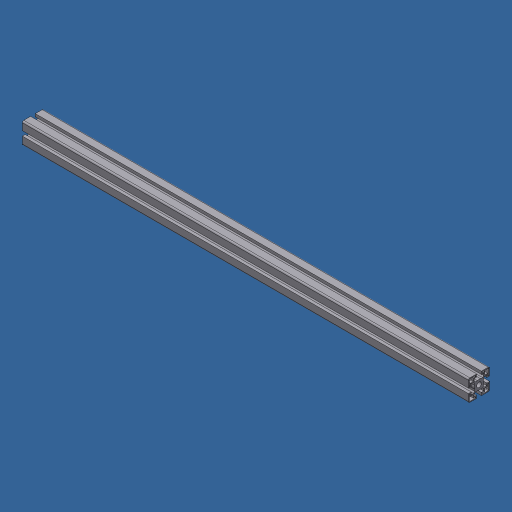
# Autodesk Inventor part: BAR, EXTRUDED ALUM, 45MMX45MM, BOSCH
Saved by Autodesk Inventor 2024.3 (Build 283343000, 343)
## iProperties
Manager: _
Category: _
RuleStatus: InUse
Shininess: 64.0
Angle Display Precision: 2
Document Length Units: 11269
Document Angle Units: 11279
Document Time Units: 11290
Document Mass Units: 11286
Document Length Units Precision: 3
Document Angle Units Precision: 2
Part Number: BAR, EXTRUDED ALUM, 45MMX45MM, BOSCH
Material: Aluminum, 6061-T6
Document SubType Name: Modeling
Created: 2019-07-31
Designer: -
Manufacturer: Standard
Standards Organization: Custom
Checked By: 00
Engr Approved By: R
User Status: Work In Proces
Description: BAR, EXTRUDED ALUM, 45MMX45MM, BOSCH
Density: 2.71 g/cm^3
Mass: 2044.87 g
Surface Area: 5623.1 cm^2
Volume: 754.565 cm^3
Mfg Approved By: -
Appearance: Aluminum (Flat)
BeforeDocSave0: Mass
BeforeDocSave1: PartFinishTrigger
Density: 0.0
Volumn: 0.0
Area: 0.0
PropertySet Name: Model Information
Control State: 0
Master: False
Checked Out: False
CN_MASS: 5.93
CN_SERVICEABLE: _
CL_runCount: 0
FIRST_DESCRIPTION: _
SECOND_DESCRIPTION: _
THIRD_DESCRIPTION: _
Revision Number: A
Subject: _
Author: -
Keywords: -
Autodesk Inventor part; units mm, degrees
ref_plane "YZ Plane" through (0, 0, 0) normal (1, 0, 0) x (0, 1, 0)
ref_plane "XZ Plane" through (0, 0, 0) normal (0, 1, 0) x (-1, 0, 0)
ref_plane "Work Plane1" through (-188.9125, 0, 0) normal (1, 0, 0) x (0, 1, 0)
sketch "Sketch1" plane through (-188.9125, 0, 0) normal (1, 0, 0) x (0, 1, 0)
  line L0 (-22.5, -5) -> (-16.5, -5) projected
  line L1 (-16.5, -5) -> (-16.5, -10.05) projected
  line L2 (-16.5, -10.05) -> (-11.9175, -10.05) projected
  line L3 (-11.9175, -10.05) -> (-9.3675, -7.5) projected
  line L4 (-9.3675, -7.5) -> (-9.3675, -3.5) projected
  arc A0 (-9.3675, 3.5) -> (-9.3675, -3.5) centre (0, 0) ccw projected
  line L5 (-9.3675, 3.5) -> (-9.3675, 7.5) projected
  line L6 (-9.3675, 7.5) -> (-11.9175, 10.05) projected
  line L7 (-11.9175, 10.05) -> (-16.5, 10.05) projected
  line L8 (-16.5, 10.05) -> (-16.5, 5) projected
  line L9 (-22.5, 5) -> (-16.5, 5) projected
  line L10 (-22.5, 5) -> (-22.5, 19.5) projected
  arc A1 (-19.5, 22.5) -> (-22.5, 19.5) centre (-19.5, 19.5) ccw projected
  line L11 (-19.5, 22.5) -> (-5, 22.5) projected
  line L12 (-5, 22.5) -> (-5, 16.5) projected
  line L13 (-5, 16.5) -> (-10.05, 16.5) projected
  line L14 (-10.05, 16.5) -> (-10.05, 11.9175) projected
  line L15 (-10.05, 11.9175) -> (-7.5, 9.3675) projected
  line L16 (-7.5, 9.3675) -> (-3.5, 9.3675) projected
  arc A2 (3.5, 9.3675) -> (-3.5, 9.3675) centre (0, 0) ccw projected
  line L17 (3.5, 9.3675) -> (7.5, 9.3675) projected
  line L18 (7.5, 9.3675) -> (10.05, 11.9175) projected
  line L19 (10.05, 11.9175) -> (10.05, 16.5) projected
  line L20 (10.05, 16.5) -> (5, 16.5) projected
  line L21 (5, 22.5) -> (5, 16.5) projected
  line L22 (5, 22.5) -> (19.5, 22.5) projected
  arc A3 (22.5, 19.5) -> (19.5, 22.5) centre (19.5, 19.5) ccw projected
  line L23 (22.5, 19.5) -> (22.5, 5) projected
  line L24 (22.5, 5) -> (16.5, 5) projected
  line L25 (16.5, 5) -> (16.5, 10.05) projected
  line L26 (16.5, 10.05) -> (11.9175, 10.05) projected
  line L27 (11.9175, 10.05) -> (9.3675, 7.5) projected
  line L28 (9.3675, 7.5) -> (9.3675, 3.5) projected
  arc A4 (9.3675, -3.5) -> (9.3675, 3.5) centre (0, 0) ccw projected
  line L29 (9.3675, -3.5) -> (9.3675, -7.5) projected
  line L30 (9.3675, -7.5) -> (11.9175, -10.05) projected
  line L31 (11.9175, -10.05) -> (16.5, -10.05) projected
  line L32 (16.5, -10.05) -> (16.5, -5) projected
  line L33 (22.5, -5) -> (16.5, -5) projected
  line L34 (22.5, -5) -> (22.5, -19.5) projected
  arc A5 (19.5, -22.5) -> (22.5, -19.5) centre (19.5, -19.5) ccw projected
  line L35 (19.5, -22.5) -> (5, -22.5) projected
  line L36 (5, -22.5) -> (5, -16.5) projected
  line L37 (5, -16.5) -> (10.05, -16.5) projected
  line L38 (10.05, -16.5) -> (10.05, -11.9175) projected
  line L39 (10.05, -11.9175) -> (7.5, -9.3675) projected
  line L40 (7.5, -9.3675) -> (3.5, -9.3675) projected
  arc A6 (-3.5, -9.3675) -> (3.5, -9.3675) centre (0, 0) ccw projected
  line L41 (-3.5, -9.3675) -> (-7.5, -9.3675) projected
  line L42 (-7.5, -9.3675) -> (-10.05, -11.9175) projected
  line L43 (-10.05, -11.9175) -> (-10.05, -16.5) projected
  line L44 (-10.05, -16.5) -> (-5, -16.5) projected
  line L45 (-5, -22.5) -> (-5, -16.5) projected
  line L46 (-5, -22.5) -> (-19.5, -22.5) projected
  arc A7 (-22.5, -19.5) -> (-19.5, -22.5) centre (-19.5, -19.5) ccw projected
  line L47 (-22.5, -19.5) -> (-22.5, -5) projected
  arc A8 (0, 5) -> (0, -5) centre (0, 0) ccw projected
  arc A9 (0, -5) -> (0, 5) centre (0, 0) ccw projected
  arc A10 (13.05, -12.05) -> (12.05, -13.05) centre (13.05, -13.05) ccw projected
  line L48 (12.05, -13.05) -> (12.05, -18.5) projected
  line L49 (12.05, -18.5) -> (7, -18.5) projected
  line L50 (7, -18.5) -> (7, -20.5) projected
  line L51 (7, -20.5) -> (19.5, -20.5) projected
  arc A11 (19.5, -20.5) -> (20.5, -19.5) centre (19.5, -19.5) ccw projected
  line L52 (20.5, -19.5) -> (20.5, -7) projected
  line L53 (20.5, -7) -> (18.5, -7) projected
  line L54 (18.5, -7) -> (18.5, -12.05) projected
  line L55 (18.5, -12.05) -> (13.05, -12.05) projected
  arc A12 (-20.5, -19.5) -> (-19.5, -20.5) centre (-19.5, -19.5) ccw projected
  line L56 (-19.5, -20.5) -> (-7, -20.5) projected
  line L57 (-7, -20.5) -> (-7, -18.5) projected
  line L58 (-7, -18.5) -> (-12.05, -18.5) projected
  line L59 (-12.05, -18.5) -> (-12.05, -13.05) projected
  arc A13 (-12.05, -13.05) -> (-13.05, -12.05) centre (-13.05, -13.05) ccw projected
  line L60 (-13.05, -12.05) -> (-18.5, -12.05) projected
  line L61 (-18.5, -12.05) -> (-18.5, -7) projected
  line L62 (-18.5, -7) -> (-20.5, -7) projected
  line L63 (-20.5, -7) -> (-20.5, -19.5) projected
  arc A14 (-19.5, 20.5) -> (-20.5, 19.5) centre (-19.5, 19.5) ccw projected
  line L64 (-20.5, 19.5) -> (-20.5, 7) projected
  line L65 (-20.5, 7) -> (-18.5, 7) projected
  line L66 (-18.5, 7) -> (-18.5, 12.05) projected
  line L67 (-18.5, 12.05) -> (-13.05, 12.05) projected
  arc A15 (-13.05, 12.05) -> (-12.05, 13.05) centre (-13.05, 13.05) ccw projected
  line L68 (-12.05, 13.05) -> (-12.05, 18.5) projected
  line L69 (-12.05, 18.5) -> (-7, 18.5) projected
  line L70 (-7, 18.5) -> (-7, 20.5) projected
  line L71 (-7, 20.5) -> (-19.5, 20.5) projected
  line L72 (7, 18.5) -> (12.05, 18.5) projected
  line L73 (12.05, 18.5) -> (12.05, 13.05) projected
  arc A16 (12.05, 13.05) -> (13.05, 12.05) centre (13.05, 13.05) ccw projected
  line L74 (13.05, 12.05) -> (18.5, 12.05) projected
  line L75 (18.5, 12.05) -> (18.5, 7) projected
  line L76 (18.5, 7) -> (20.5, 7) projected
  line L77 (20.5, 7) -> (20.5, 19.5) projected
  arc A17 (20.5, 19.5) -> (19.5, 20.5) centre (19.5, 19.5) ccw projected
  line L78 (19.5, 20.5) -> (7, 20.5) projected
  line L79 (7, 20.5) -> (7, 18.5) projected
  line L80 (5, -22.5) -> (19.5, -22.5)
  line L81 (19.5, -20.5) -> (7, -20.5)
  line L82 (7, -20.5) -> (7, -18.5)
  line L83 (7, -18.5) -> (12.05, -18.5)
  line L84 (12.05, -18.5) -> (12.05, -13.05)
  line L85 (18.5, -12.05) -> (13.05, -12.05)
  line L86 (18.5, -12.05) -> (18.5, -7)
  line L87 (18.5, -7) -> (20.5, -7)
  line L88 (20.5, -7) -> (20.5, -19.5)
  line L89 (22.5, -19.5) -> (22.5, -5)
  line L90 (22.5, -5) -> (16.5, -5)
  line L91 (11.9175, -10.05) -> (16.5, -10.05)
  line L92 (16.5, -10.05) -> (16.5, -5)
  line L93 (11.9175, -10.05) -> (9.3675, -7.5)
  line L94 (7.5, -9.3675) -> (10.05, -11.9175)
  line L95 (10.05, -11.9175) -> (10.05, -16.5)
  line L96 (10.05, -16.5) -> (5, -16.5)
  line L97 (5, -22.5) -> (5, -16.5)
  line L98 (7.5, -9.3675) -> (3.5, -9.3675)
  line L99 (9.3675, -7.5) -> (9.3675, -3.5)
  line L100 (9.3675, 3.5) -> (9.3675, 7.5)
  line L101 (9.3675, 7.5) -> (11.9175, 10.05)
  line L102 (11.9175, 10.05) -> (16.5, 10.05)
  line L103 (16.5, 10.05) -> (16.5, 5)
  line L104 (16.5, 5) -> (22.5, 5)
  line L105 (22.5, 5) -> (22.5, 19.5)
  line L106 (20.5, 19.5) -> (20.5, 7)
  line L107 (18.5, 7) -> (20.5, 7)
  line L108 (18.5, 7) -> (18.5, 12.05)
  line L109 (18.5, 12.05) -> (13.05, 12.05)
  line L110 (12.05, 13.05) -> (12.05, 18.5)
  line L111 (12.05, 18.5) -> (7, 18.5)
  line L112 (7, 18.5) -> (7, 20.5)
  line L113 (7, 20.5) -> (19.5, 20.5)
  line L114 (19.5, 22.5) -> (5, 22.5)
  line L115 (5, 22.5) -> (5, 16.5)
  line L116 (5, 16.5) -> (10.05, 16.5)
  line L117 (10.05, 16.5) -> (10.05, 11.9175)
  line L118 (10.05, 11.9175) -> (7.5, 9.3675)
  line L119 (7.5, 9.3675) -> (3.5, 9.3675)
  line L120 (-3.5, 9.3675) -> (-7.5, 9.3675)
  line L121 (-7.7267, 9.5942) -> (-10.05, 11.9175)
  line L122 (-10.05, 11.9175) -> (-10.05, 16.5)
  line L123 (-10.05, 16.5) -> (-5, 16.5)
  line L124 (-5, 16.5) -> (-5, 22.5)
  line L125 (-19.5, 22.5) -> (-5, 22.5)
  line L126 (-7, 20.5) -> (-19.5, 20.5)
  line L127 (-7, 20.5) -> (-7, 18.5)
  line L128 (-7, 18.5) -> (-12.05, 18.5)
  line L129 (-12.05, 18.5) -> (-12.05, 13.05)
  line L130 (-13.05, 12.05) -> (-18.5, 12.05)
  line L131 (-18.5, 12.05) -> (-18.5, 7)
  line L132 (-18.5, 7) -> (-20.5, 7)
  line L133 (-20.5, 7) -> (-20.5, 19.5)
  line L134 (-22.5, 19.5) -> (-22.5, 5)
  line L135 (-22.5, 5) -> (-16.5, 5)
  line L136 (-16.5, 5) -> (-16.5, 10.05)
  line L137 (-11.9175, 10.05) -> (-16.5, 10.05)
  line L138 (-11.9175, 10.05) -> (-9.3675, 7.5)
  line L139 (-9.3675, 7.5) -> (-9.3675, 3.5)
  line L140 (-9.3675, -3.5) -> (-9.3675, -7.5)
  line L141 (-9.3675, -7.5) -> (-11.9175, -10.05)
  line L142 (-11.9175, -10.05) -> (-16.5, -10.05)
  line L143 (-16.5, -10.05) -> (-16.5, -5)
  line L144 (-16.5, -5) -> (-22.5, -5)
  line L145 (-22.5, -5) -> (-22.5, -19.5)
  line L146 (-20.5, -7) -> (-20.5, -19.5)
  line L147 (-20.5, -7) -> (-18.5, -7)
  line L148 (-18.5, -7) -> (-18.5, -12.05)
  line L149 (-18.5, -12.05) -> (-13.05, -12.05)
  line L150 (-12.05, -13.05) -> (-12.05, -18.5)
  line L151 (-12.05, -18.5) -> (-7, -18.5)
  line L152 (-7, -18.5) -> (-7, -20.5)
  line L153 (-7, -20.5) -> (-19.5, -20.5)
  line L154 (-19.5, -22.5) -> (-5, -22.5)
  line L155 (-5, -22.5) -> (-5, -16.5)
  line L156 (-5, -16.5) -> (-10.05, -16.5)
  line L157 (-10.05, -16.5) -> (-10.05, -11.9175)
  line L158 (-7.5, -9.3675) -> (-10.05, -11.9175)
  line L159 (-7.5, -9.3675) -> (-3.5, -9.3675)
  arc A18 (-20.5, -19.5) -> (-19.5, -20.5) centre (-19.5, -19.5) ccw
  arc A19 (-22.5, -19.5) -> (-19.5, -22.5) centre (-19.5, -19.5) ccw
  arc A20 (-12.05, -13.05) -> (-13.05, -12.05) centre (-13.05, -13.05) ccw
  circle A21 centre (0, 0) radius 5
  arc A22 (-13.05, 12.05) -> (-12.05, 13.05) centre (-13.05, 13.05) ccw
  arc A23 (-19.5, 20.5) -> (-20.5, 19.5) centre (-19.5, 19.5) ccw
  arc A24 (-19.5, 22.5) -> (-22.5, 19.5) centre (-19.5, 19.5) ccw
  arc A25 (12.05, 13.05) -> (13.05, 12.05) centre (13.05, 13.05) ccw
  arc A26 (20.5, 19.5) -> (19.5, 20.5) centre (19.5, 19.5) ccw
  arc A27 (22.5, 19.5) -> (19.5, 22.5) centre (19.5, 19.5) ccw
  arc A28 (13.05, -12.05) -> (12.05, -13.05) centre (13.05, -13.05) ccw
  arc A29 (19.5, -20.5) -> (20.5, -19.5) centre (19.5, -19.5) ccw
  arc A30 (19.5, -22.5) -> (22.5, -19.5) centre (19.5, -19.5) ccw
  arc A31 (-3.5, -9.3675) -> (3.5, -9.3675) centre (0, 0) ccw
  arc A32 (9.3675, -3.5) -> (9.3675, 3.5) centre (0, 0) ccw
  arc A33 (3.5, 9.3675) -> (-3.5, 9.3675) centre (0, 0) ccw
  arc A34 (-9.3675, 3.5) -> (-9.3675, -3.5) centre (0, 0) ccw
  constraints: 160 end point, 68 equal length, 37 point on circle, 24 tangent, 16 centre point, 14 coincident, 12 concentric, 12 perpendicular, 1 point on line, 1 vertical alignment, 2 other
extrude "BOSCH, 45X45" add sketch "Sketch1" along normal blind 945
